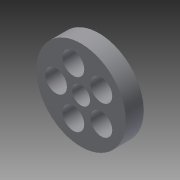
# Autodesk Inventor part: ротор редуктора
Saved by Autodesk Inventor 2013 (Build 170138000, 138)
## iProperties
Created: 2014-04-30
Part Number: ротор редуктора
Material: Типовые
Document SubType Name: Modeling
Designer: HP1
Density: 1 g/cm^3
Mass: 13.0046 g
Surface Area: 64.0225 cm^2
Volume: 13.0046 cm^3
Author: HP1
Autodesk Inventor part; units mm, degrees
ref_plane "YZ Plane" through (0, 0, 0) normal (1, 0, 0) x (0, 1, 0)
ref_plane "XZ Plane" through (0, 0, 0) normal (0, 1, 0) x (-1, 0, 0)
ref_plane "XY Plane" through (0, 0, 0) normal (0, 0, 1) x (1, 0, 0)
sketch "Эскиз1" plane through (0, 0, 0) normal (0, 1, 0) x (-1, 0, 0)
  circle A0 centre (0, 0) radius 5
  circle A1 centre (0, 0) radius 25
  circle A2 centre (14, 0) radius 6.1
  circle A3 centre (4.3262, 13.3148) radius 6.1
  circle A4 centre (-11.3262, 8.229) radius 6.1
  circle A5 centre (-11.3262, -8.229) radius 6.1
  circle A6 centre (4.3262, -13.3148) radius 6.1
  dimension "d2" = 10
  dimension "d3" = 50
  dimension "d4" = 12.2
  dimension "d5" = 14
  dimension "d6" = 360
  constraints: 7 centre point, 11 other
  measures "d2" diameter of A0
  measures "d3" diameter of A1
  measures "d4" diameter of A2
  measures "d5" distance of A1.centre A2.centre
extrude "Выдавливание1" add sketch "Эскиз1" along normal blind 10
